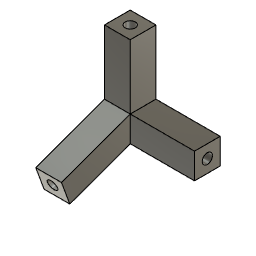
Collin_Corner Connector 1 v2 v1 (Autodesk Fusion 360 design; units mm, degrees)
Autodesk Fusion 360 part; units mm, degrees
sketch "Sketch1" plane through (0, 0, 0) normal (0, 1, 0) x (1, 0, 0)
  line L0 (0, 0) -> (14, 0)
  line L1 (14, 0) -> (14, -4)
  line L2 (14, -4) -> (0, -4)
  line L3 (0, -4) -> (0, 0)
  line L4 (0, 0) -> (4, 0)
  line L5 (4, 0) -> (4, -14)
  line L6 (4, -14) -> (0, -14)
  line L7 (0, -14) -> (0, 0)
  dimension "d1" = 4
  dimension "d2" = 4
  dimension "d3" = 14
  dimension "d4" = 14
  constraint horizontal L0
  constraint vertical L1
  constraint horizontal L2
  constraint vertical L3
  constraint coincident L0.start L3.end
  constraint horizontal L4
  constraint vertical L5
  constraint horizontal L6
  constraint vertical L7
  measures "d1" distance of L0.start L4.end
  measures "d2" distance of L0.start L2.end
  measures "d3" distance of L1 L7
  measures "d4" distance of L4 L6
extrude "Extrude1" add sketch "Sketch1" along normal blind 4
sketch "Sketch2" plane through (0, 0, 14) normal (0, 0, 1) x (-1, 0, 0)
  line L0 (0, 0) -> (-4, 0)
  line L1 (-4, 0) -> (-4, -4)
  line L2 (-4, -4) -> (0, -4)
  line L3 (0, -4) -> (0, 0)
  circle A0 centre (-2, -2) radius 0.8
  dimension "BORE" = 1.6
  dimension "d8" = 2
  dimension "d9" = 2
  measures "BORE" diameter of A0
  measures "d8" distance of L2 A0.centre
  measures "d9" distance of L3 A0.centre
extrude "Extrude2" cut sketch "Sketch2" against normal blind 10 contours A0
sketch "Sketch3" plane through (14, 0, 0) normal (1, 0, 0) x (0, 1, 0)
  line L0 (0, 4) -> (0, 0)
  line L1 (0, 0) -> (4, 0)
  line L2 (4, 0) -> (4, 4)
  line L3 (4, 4) -> (0, 4)
  circle A0 centre (2, 2) radius 0.8
  dimension "d12" = 1.6
  dimension "d13" = 2
  dimension "d14" = 2
  measures "d12" diameter of A0
  measures "d13" distance of L1 A0.centre
  measures "d14" distance of L0 A0.centre
extrude "Extrude3" cut sketch "Sketch3" against normal blind 10 contours A0
ref_plane "WorkPlane1" through (12.125, 0, 0) normal (0, -0.939693, -0.34202) x (1, 0, 0)
sketch "Sketch4" plane through (12.125, 0, 0) normal (0, -0.939693, -0.34202) x (1, 0, 0)
  line L0 (-8.125, 13.1557) -> (-12.125, 13.1557)
  line L1 (-12.125, 13.1557) -> (-12.125, 0)
  line L2 (-12.125, 0) -> (1.875, 0)
  line L3 (1.875, 0) -> (1.875, 3.7588)
  line L4 (1.875, 3.7588) -> (-8.125, 3.7588)
  line L5 (-8.125, 3.7588) -> (-8.125, 13.1557)
  line L6 (-8.125, 3.7588) -> (-12.125, 3.7588)
  line L7 (-12.125, 3.7588) -> (-12.125, 0)
  line L8 (-12.125, 0) -> (-8.125, 0)
  line L9 (-8.125, 0) -> (-8.125, 3.7588)
  circle A0 centre (-10.125, 2) radius 0.8
  dimension "d18" = 1.6
  dimension "d19" = 2
  dimension "d20" = 2
  constraint horizontal L6
  constraint vertical L7
  constraint horizontal L8
  constraint vertical L9
  constraint coincident L1.end L2.start
  constraint coincident L4.end L5.start
  measures "d18" diameter of A0
  measures "d19" distance of L7 A0.centre
  measures "d20" distance of L8 A0.centre
extrude "Extrude4" add sketch "Sketch4" along normal blind 10 contours L1 L2 L6 L7 L8 L9
extrude "Extrude5" add sketch "Sketch4" along normal up to surface contours L1 L2 L6 L7 L8 L9 end surface through (0, 0, 0) normal (0, -1, 0) offset 0
equation "d12 = BORE"
equation "d18 = BORE"
